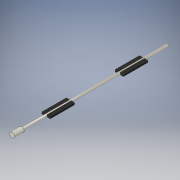
# Autodesk Inventor part: Rod
Saved by Autodesk Inventor 2018 (Build 220112000, 112)
## iProperties
Created: 2021-03-16
Part Number: Rod
Material: Generic
Document SubType Name: Modeling
Designer: Patel
Density: 1 g/cm^3
Appearance: Default
Author: Patel
Autodesk Inventor part; units mm, degrees
ref_plane "YZ Plane" through (0, 0, 0) normal (1, 0, 0) x (0, 1, 0)
ref_plane "XZ Plane" through (0, 0, 0) normal (0, 1, 0) x (-1, 0, 0)
ref_plane "XY Plane" through (0, 0, 0) normal (0, 0, 1) x (1, 0, 0)
sketch "Sketch1" plane through (0, 0, 0) normal (0, 0, 1) x (1, 0, 0)
  circle A0 centre (0, 0) radius 2.5
  dimension "d0" = 5
  constraints: 1 centre point, 1 coincident
  measures "d0" diameter of A0
extrude "Extrusion1" add sketch "Sketch1" against normal blind 300
sketch "Sketch2" plane through (0, 0, 0) normal (0, 1, 0) x (-1, 0, 0)
  line L0 (1.5, -50) -> (8.5, -50)
  line L1 (8.5, -50) -> (8.5, -100)
  line L2 (8.5, -100) -> (1.5, -100)
  line L3 (1.5, -100) -> (1.5, -50)
  line L4 (1.5, -250) -> (8.5, -250)
  line L5 (8.5, -250) -> (8.5, -200)
  line L6 (8.5, -200) -> (1.5, -200)
  line L7 (1.5, -200) -> (1.5, -250)
  point P0 (0, 0)
  dimension "d3" = 7
  dimension "d4" = 50
  dimension "d5" = 7
  dimension "d6" = 50
  dimension "d7" = 0
  dimension "d8" = 150
  dimension "d9" = 8.5
  dimension "d10" = 50
  constraints: 16 end point, 4 parallel, 2 horizontal, 2 perpendicular
  measures "d3" distance of L1.end L2.end
  measures "d4" distance of L0.end L1.end
  measures "d5" distance of L6.end L5.end
  measures "d6" distance of L5.end L4.end
  measures "d7" distance between parallel lines of L1 L5
  measures "d8" distance between parallel lines of L0 L6
  measures "d9" distance from line of point (0, 0) L1
  measures "d10" distance from line of point (0, 0) L0
extrude "Extrusion2" add sketch "Sketch2" along normal mid plane 4
mirror "Mirror1" about plane through (0, 0, 0) normal (1, 0, 0) of "Extrusion2"
sketch "Sketch3" plane through (0, 0, 0) normal (0, 0, 1) x (1, 0, 0)
  circle A0 centre (0, 0) radius 5
  dimension "d13" = 10
  constraints: 1 centre point, 1 coincident
  measures "d13" diameter of A0
extrude "Extrusion3" add sketch "Sketch3" along normal blind 20
body "Solid1"
